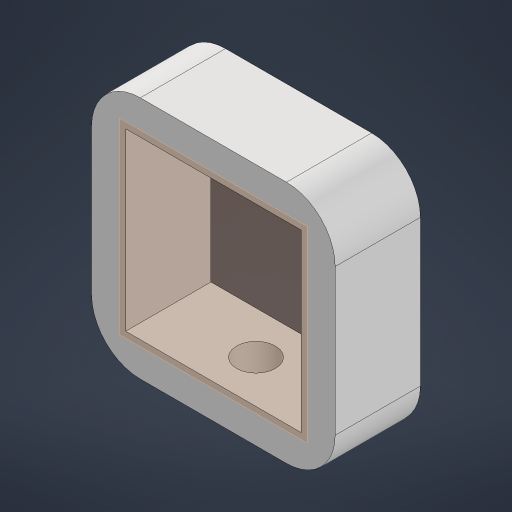
# Autodesk Inventor part: Tap_zigu
Saved by Autodesk Inventor 2024.2 (Build 282272000, 272)
## iProperties
Created: 2024-02-10
Part Number: Tap_zigu
Material: 一般
Document SubType Name: Modeling
Designer: Hanaoka
Density: 1 g/cm^3
Appearance: 既定
Author: Hanaoka
Autodesk Inventor part; units mm, degrees
ref_plane "YZ Plane" through (0, 0, 0) normal (1, 0, 0) x (0, 1, 0)
ref_plane "XZ Plane" through (0, 0, 0) normal (0, 1, 0) x (-1, 0, 0)
ref_plane "XY Plane" through (0, 0, 0) normal (0, 0, 1) x (1, 0, 0)
ref_plane "作業平面1" through (26.683, 7.3716, 0.277) normal (0, 0, 1) x (0, -1, 0)
sketch "スケッチ1" plane through (26.683, 7.3716, 0.277) normal (0, 0, 1) x (0, -1, 0)
  arc A0 (0.9652, -1.8217) -> (0.7443, -1.8564) centre (0.9303, -2.3204) ccw projected
  arc A1 (0.7443, 1.8564) -> (0.7443, -1.8564) centre (0, 0) ccw projected
  arc A2 (0.7443, 1.8564) -> (0.9652, 1.8217) centre (0.9303, 2.3204) ccw projected
  arc A3 (1.5, 1.3229) -> (0.9652, 1.8217) centre (1, 1.3229) ccw projected
  line L0 (1.5, 1.3229) -> (1.5, -1.3229) projected
  arc A4 (0.9652, -1.8217) -> (1.5, -1.3229) centre (1, -1.3229) ccw projected
  arc A5 (2, -3.5) -> (3.5, -2) centre (2, -2) ccw projected
  line L1 (3.5, -2) -> (3.5, 2) projected
  arc A6 (3.5, 2) -> (2, 3.5) centre (2, 2) ccw projected
  line L2 (2, 3.5) -> (-2, 3.5) projected
  arc A7 (-2, 3.5) -> (-3.5, 2) centre (-2, 2) ccw projected
  line L3 (-3.5, 2) -> (-3.5, -2) projected
  arc A8 (-3.5, -2) -> (-2, -3.5) centre (-2, -2) ccw projected
  line L4 (-2, -3.5) -> (2, -3.5) projected
  line L5 (5, -5) -> (-5, -5)
  line L6 (-5, -5) -> (-5, 5)
  line L7 (-5, 5) -> (5, 5)
  line L8 (5, 5) -> (5, -5)
  line L9 (5, -5) -> (-5, 5) construction
  line L10 (-5, -5) -> (5, 5) construction
  line L11 (3.6, -3.6) -> (-3.6, -3.6)
  line L12 (-3.6, -3.6) -> (-3.6, 3.6)
  line L13 (-3.6, 3.6) -> (3.6, 3.6)
  line L14 (3.6, 3.6) -> (3.6, -3.6)
  line L15 (3.6, -3.6) -> (-3.6, 3.6) construction
  line L16 (-3.6, -3.6) -> (3.6, 3.6) construction
  point P0 (7.3716, -26.683)
  dimension "d0" = 0.1
  dimension "d1" = 10
  constraints: 24 end point, 4 midpoint, 4 parallel, 3 perpendicular, 2 horizontal, 1 point on line
  measures "d0" distance between parallel lines of L3 L12
  measures "d1" distance of L5.end L6.end
extrude "押し出し1" add sketch "スケッチ1" against normal blind 3.5 contours L5 L6 L7 L8
fillet "フィレット1" radius 2 4 edges at (31.683, 12.3716, -1.473) (21.683, 12.3716, -1.473) (21.683, 2.3716, -1.473) (31.683, 2.3716, -1.473)
sketch "スケッチ3" plane through (23.683, 2.3716, 0.277) normal (0, -1, 0) x (1, 0, 0)
  line L0 (6, 0) -> (6, -3.5) projected
  line L1 (0, 0) -> (6, 0) projected
  line L2 (0, -3.5) -> (0, 0) projected
  line L3 (6, -3.5) -> (0, -3.5) projected
  line L4 (8, -3.5) -> (6, -3.5) projected
  line L5 (0, 0) -> (6, -3.5) construction
  circle A0 centre (3, -1.75) radius 0.8
  point P0 (-23.683, -0.277)
  dimension "d11" = 1.6
  constraints: 2 end point, 1 centre point, 1 coincident, 1 midpoint
  measures "d11" diameter of A0
extrude "押し出し3" cut sketch "スケッチ3" against normal blind 3.5 contours A0
